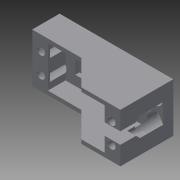
# Autodesk Inventor part: forearm_anti_axe
Saved by Autodesk Inventor 2015 (Build 190159000, 159)
## iProperties
Created: 2015-09-27
Part Number: forearm_anti_axe
Material: Générique
Document SubType Name: Modeling
Designer: astralien3000
Density: 1 g/cm^3
Appearance: Par défaut
Author: astralien3000
Autodesk Inventor part; units mm, degrees
ref_plane "YZ Plane" through (0, 0, 0) normal (1, 0, 0) x (0, 1, 0)
ref_plane "XZ Plane" through (0, 0, 0) normal (0, 1, 0) x (-1, 0, 0)
ref_plane "XY Plane" through (0, 0, 0) normal (0, 0, 1) x (1, 0, 0)
sketch "Esquisse1" plane through (0, 0, 0) normal (0, 1, 0) x (-1, 0, 0)
  line L0 (21, 10.5) -> (-21, 10.5)
  line L1 (-21, 10.5) -> (-21, -10.5)
  line L2 (-21, -10.5) -> (21, -10.5)
  line L3 (21, -10.5) -> (21, 10.5)
  line L4 (29, 12.5) -> (-29, 12.5)
  line L5 (-29, 12.5) -> (-29, -12.5)
  line L6 (-29, -12.5) -> (29, -12.5)
  line L7 (29, -12.5) -> (29, 12.5)
  point P0 (0, 0)
  dimension "d0" = 21
  dimension "d1" = 10.5
  dimension "d2" = 42
  dimension "d3" = 21
  dimension "d4" = 2
  dimension "d5" = 2
  dimension "d6" = 8
  dimension "d7" = 8
  constraints: 16 end point, 4 parallel, 2 horizontal, 2 perpendicular
  measures "d0" distance between parallel lines of L0 L2
  measures "d1" distance from line of L2 point (0, 0)
  measures "d2" distance between parallel lines of L1 L3
  measures "d3" distance from line of L1 point (0, 0)
  measures "d4" distance between parallel lines of L0 L4
  measures "d5" distance between parallel lines of L6 L2
  measures "d6" distance between parallel lines of L7 L3
  measures "d7" distance between parallel lines of L5 L1
extrude "Extrusion1" add sketch "Esquisse1" along normal blind 28
sketch "Esquisse2" plane through (0, 28, 0) normal (0, 1, 0) x (1, 0, 0)
  line L0 (-29, -12.5) -> (29, -12.5)
  line L1 (29, -12.5) -> (29, 12.5)
  line L2 (29, 12.5) -> (-29, 12.5)
  line L3 (-29, 12.5) -> (-29, -12.5)
  point P0 (0, 0)
  constraints: 8 end point, 2 coincident, 2 parallel, 1 horizontal, 1 perpendicular
extrude "Extrusion2" add sketch "Esquisse2" along normal blind 5
sketch "Esquisse3" plane through (0, 0, 0) normal (0, -1, 0) x (1, 0, 0)
  line L0 (-28, 10.5) -> (-21, 0) construction
  line L1 (-21, 0) -> (-28, -10.5) construction
  line L2 (-21, -10.5) -> (-28, 0) construction
  line L3 (-28, 0) -> (-21, 10.5) construction
  line L4 (21, 10.5) -> (28, 0) construction
  line L5 (21, -10.5) -> (28, 0) construction
  line L6 (28, -10.5) -> (21, 0) construction
  line L7 (21, 0) -> (28, 10.5) construction
  circle A0 centre (24.5, 5.25) radius 2
  circle A1 centre (24.5, -5.25) radius 2
  circle A2 centre (-24.5, 5.25) radius 2
  circle A3 centre (-24.5, -5.25) radius 2
  line L8 (-21, 10.5) -> (-28, 10.5)
  line L9 (-28, 10.5) -> (-28, -10.5)
  line L10 (-28, -10.5) -> (-21, -10.5)
  line L11 (-21, -10.5) -> (-21, 10.5)
  line L12 (28, 10.5) -> (21, 10.5)
  line L13 (21, 10.5) -> (21, -10.5)
  line L14 (21, -10.5) -> (28, -10.5)
  line L15 (28, -10.5) -> (28, 10.5)
  line L16 (21, 10.5) -> (21, -10.5) projected
  line L17 (21, -10.5) -> (-21, -10.5) projected
  line L18 (-21, 10.5) -> (21, 10.5) projected
  line L19 (-21, -10.5) -> (-21, 10.5) projected
  point P0 (0, 0)
  dimension "d12" = 4
  dimension "d13" = 4
  dimension "d14" = 4
  dimension "d15" = 4
  dimension "d25" = 7
  dimension "d26" = 7
  constraints: 32 end point, 8 midpoint, 6 parallel, 5 collinear, 4 centre point, 2 horizontal, 2 perpendicular, 1 coincident, 1 point on line
  measures "d12" diameter of A2
  measures "d13" diameter of A3
  measures "d14" diameter of A0
  measures "d15" diameter of A1
  measures "d25" distance between parallel lines of L13 L15
  measures "d26" distance between parallel lines of L11 L9
extrude "Extrusion3" cut sketch "Esquisse3" against normal through all contours A0 | A1 | A2 | A3
sketch "Esquisse4" plane through (0, 28, 0) normal (0, -1, 0) x (1, 0, 0)
  line L0 (-21, 10.5) -> (10, 10.5)
  line L1 (10, 10.5) -> (10, -10.5)
  line L2 (10, -10.5) -> (-21, -10.5)
  line L3 (-21, -10.5) -> (-21, 10.5)
  line L4 (21, -10.5) -> (-21, -10.5) projected
  circle A0 centre (10, 0) radius 3.5
  line L5 (21, 10.5) -> (21, -10.5) projected
  point P0 (0, 0)
  dimension "d19" = 7
  dimension "d50" = 11
  constraints: 8 end point, 2 parallel, 1 centre point, 1 coincident, 1 collinear, 1 horizontal, 1 midpoint, 1 perpendicular
  measures "d19" diameter of A0
  measures "d50" distance between parallel lines of L5 L1
extrude "Extrusion4" cut sketch "Esquisse4" against normal through all contours A0 L1 | L1 A0
chamfer "Chanfrein1" distance 3 angle 45 1 edges at (6.5, 28, 0)
sketch "Esquisse5" plane through (-29, 0, 12.5) normal (0, 0, 1) x (1, 0, 0)
  line L0 (0, 0) -> (25, 0)
  line L1 (25, 0) -> (25, 19)
  line L2 (25, 19) -> (0, 19)
  line L3 (0, 19) -> (0, 0)
  line L4 (25, 0) -> (58, 0)
  line L5 (58, 0) -> (58, 6)
  line L6 (58, 6) -> (25, 6)
  line L7 (25, 6) -> (25, 0)
  line L8 (25, 19) -> (38, 6)
  point P0 (29, 0)
  dimension "d27" = 19
  dimension "d29" = 6
  dimension "d30" = 45
  dimension "d33" = 20
  constraints: 18 end point, 4 parallel, 2 horizontal, 2 perpendicular, 1 coincident, 1 point on line
  measures "d27" distance of L2.end L0.start
  measures "d29" distance of L4.end L5.end
  measures "d30" angle of L8 L1
  measures "d33" distance of L5.end L8.end
extrude "Extrusion5" cut sketch "Esquisse5" against normal through all
sketch "Esquisse6" plane through (0, 33, 0) normal (0, 1, 0) x (1, 0, 0)
  circle A0 centre (-24.5, -5.25) radius 4
  circle A1 centre (-24.5, 5.25) radius 4
  circle A2 centre (24.5, -5.25) radius 4
  circle A3 centre (24.5, 5.25) radius 4
  circle A4 centre (24.5, 5.25) radius 2 projected
  circle A5 centre (24.5, -5.25) radius 2 projected
  circle A6 centre (-24.5, -5.25) radius 2 projected
  circle A7 centre (-24.5, 5.25) radius 2 projected
  point P0 (0, 0)
  dimension "d34" = 8
  dimension "d35" = 8
  dimension "d36" = 8
  dimension "d37" = 8
  constraints: 4 centre point, 4 concentric
  measures "d34" diameter of A0
  measures "d35" diameter of A1
  measures "d36" diameter of A2
  measures "d37" diameter of A3
extrude "Extrusion6" cut sketch "Esquisse6" against normal blind 13
sketch "Esquisse7" plane through (29, 33, 12.5) normal (1, 0, 0) x (0, 0, -1)
  line L0 (7.5, -27) -> (17.5, -27)
  line L1 (17.5, -27) -> (17.5, -5)
  line L2 (17.5, -5) -> (7.5, -5)
  line L3 (7.5, -5) -> (7.5, -27)
  line L4 (0, -27) -> (25, -27) projected
  line L5 (15.8135, -5) -> (9.1865, -5) projected
  line L6 (17.5, -27) -> (15.5, -27)
  line L7 (15.5, -27) -> (15.5, -17)
  line L8 (15.5, -17) -> (17.5, -17)
  line L9 (17.5, -17) -> (17.5, -27)
  line L10 (7.5, -27) -> (9.5, -27)
  line L11 (9.5, -27) -> (9.5, -17)
  line L12 (9.5, -17) -> (7.5, -17)
  line L13 (7.5, -17) -> (7.5, -27)
  point P0 (12.5, -33)
  dimension "d40" = 10
  dimension "d41" = 5
  dimension "d44" = 6
  dimension "d45" = 3
  dimension "d46" = 10
  constraints: 24 end point, 6 parallel, 3 horizontal, 3 perpendicular, 2 collinear, 1 point on line
  measures "d40" distance between parallel lines of L1 L3
  measures "d41" distance from line of point (12.5, -33) L3
  measures "d44" distance between parallel lines of L7 L11
  measures "d45" distance from line of point (12.5, -33) L11
  measures "d46" distance between parallel lines of L4 L12
extrude "Extrusion7" cut sketch "Esquisse7" against normal up to next contours L11 L12 L3 L2 L1 L8 L7 L0
chamfer "Chanfrein2" distance 2 angle 45 2 edges at (25, 16, 3) (25, 16, -3)
sketch "Esquisse8" plane through (0, 28, 0) normal (0, -1, 0) x (1, 0, 0)
  line L0 (-16, -5.5) -> (-1.5, -5.5)
  line L1 (-1.5, -5.5) -> (-1.5, 5.5)
  line L2 (-1.5, 5.5) -> (-16, 5.5)
  line L3 (-16, 5.5) -> (-16, -5.5)
  line L4 (-21, 3.3135) -> (-21, -3.3135) projected
  line L5 (-4, 10.5) -> (-21, 10.5) projected
  line L6 (-21, -10.5) -> (-4, -10.5) projected
  circle A0 centre (10, 0) radius 6.5 projected
  point P0 (0, 0)
  dimension "d51" = 5
  dimension "d52" = 5
  dimension "d53" = 5
  dimension "d54" = 5
  constraints: 8 end point, 2 parallel, 1 horizontal, 1 perpendicular
  measures "d51" distance between parallel lines of L4 L3
  measures "d52" distance between parallel lines of L5 L2
  measures "d53" distance between parallel lines of L6 L0
  measures "d54" distance edge to line of A0 L1
extrude "Extrusion8" cut sketch "Esquisse8" against normal through all contours L3 L2 L1 L0
chamfer "Chanfrein3" distance 3 angle 45 4 edges at (-8.75, 33, 5.5) (-1.5, 33, 0) (-8.75, 33, -5.5) (-16, 33, 0)
equation "\"d1\" = 0.5 * d0"
equation "\"d3\" = 0.5 * d2"
equation "\"d13\" = d12"
equation "\"d14\" = d12"
equation "\"d15\" = d12"
equation "\"d35\" = d34"
equation "\"d36\" = d34"
equation "\"d37\" = d34"
equation "\"d41\" = 0.5 * d40"
equation "\"d45\" = 0.5 * d44"
